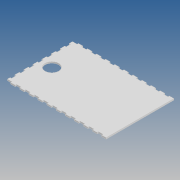
# Autodesk Inventor part: 000.104 - Cap
Saved by Autodesk Inventor 2020 (Build 240168000, 168)
## iProperties
Created: 2021-06-28
Part Number: 000.104 - Cap
Material: Типовые
Document SubType Name: Modeling
Designer: Петров Иван
Mass: 93.6094 g
Surface Area: 653.89 cm^2
Volume: 93.6094 cm^3
Density: 1 g/cm^3
Appearance: По умолчанию
Author: Петров Иван
Autodesk Inventor part; units mm, degrees
ref_plane "YZ Plane" through (0, 0, 0) normal (1, 0, 0) x (0, 1, 0)
ref_plane "XZ Plane" through (0, 0, 0) normal (0, 1, 0) x (-1, 0, 0)
ref_plane "XY Plane" through (0, 0, 0) normal (0, 0, 1) x (1, 0, 0)
sketch "Эскиз5" plane through (0, 0, 0) normal (0, 1, 0) x (-1, 0, 0)
  line L0 (-110, 74.5) -> (110, 74.5)
  line L1 (110, 74.5) -> (110, -74.5)
  line L2 (110, -74.5) -> (-110, -74.5)
  line L3 (-110, -74.5) -> (-110, 74.5)
  line L4 (-110, 74.5) -> (110, -74.5) construction
  line L5 (110, 74.5) -> (-110, -74.5) construction
  point P0 (0, 0)
  dimension "d25" = 220
  dimension "d26" = 149
  constraints: 12 end point, 2 midpoint, 2 parallel, 1 horizontal, 1 perpendicular
  measures "d25" distance of L1.end L2.end
  measures "d26" distance of L0.end L1.end
extrude "Выдавливание5" add sketch "Эскиз5" along normal blind 3
sketch "Эскиз6" plane through (0, 3, 0) normal (0, 1, 0) x (1, 0, 0)
  line L0 (-110, 74.5) -> (-110, -74.5) projected
  line L1 (-110, -65.5) -> (-107, -65.5)
  line L2 (-107, -65.5) -> (-107, -55.5)
  line L3 (-107, -55.5) -> (-110, -55.5)
  line L4 (-110, -55.5) -> (-110, -65.5)
  line L5 (-110, -74.5) -> (110, -74.5) projected
  point P0 (0, 0)
  point P1 (-107, -74.5)
  point P2 (-110, -65.5)
  dimension "d29" = 3
  dimension "d30" = 10
  dimension "d46" = 9
  constraints: 9 end point, 2 parallel, 1 perpendicular
  measures "d29" distance of L3.end L2.end
  measures "d30" distance of L2.end L1.end
  measures "d46" distance between parallel lines of L5 L1
extrude "Выдавливание6" cut sketch "Эскиз6" against normal blind 3
pattern_linear "Прямоуг.массив6" count 7 spacing 20 along (0, 0, -1) of "Выдавливание6"
sketch "Эскиз8" plane through (0, 3, 0) normal (0, 1, 0) x (1, 0, 0)
  line L0 (-110, -74.5) -> (110, -74.5) projected
  line L1 (-110, -74.5) -> (-100, -74.5)
  line L2 (-100, -74.5) -> (-100, -71.5)
  line L3 (-100, -71.5) -> (-110, -71.5)
  line L4 (-110, -71.5) -> (-110, -74.5)
  line L5 (-107, -55.5) -> (-107, -65.5) projected
  point P0 (0, 0)
  dimension "d50" = 3
  dimension "d51" = 10
  dimension "d52" = 3
  constraints: 8 end point, 2 parallel, 1 horizontal, 1 perpendicular, 1 point on line
  measures "d50" distance of L1.end L2.end
  measures "d51" distance of L2.end L3.end
  measures "d52" distance between parallel lines of L5 L4
extrude "Выдавливание8" cut sketch "Эскиз8" against normal blind 3
pattern_linear "Прямоуг.массив7" count 11 spacing 20 along (1, 0, 0) of "Выдавливание8"
mirror "Зеркальное отражение2" about plane through (0, 0, 0) normal (0, 0, 1) of "Выдавливание8", "Прямоуг.массив7"
sketch "Эскиз9" plane through (0, 3, 0) normal (0, 1, 0) x (1, 0, 0)
  circle A0 centre (-83.8133, 0) radius 15
  point P0 (0, 0)
  dimension "d58" = 30
  constraints: 1 centre point
  measures "d58" diameter of A0
extrude "Выдавливание9" cut sketch "Эскиз9" against normal blind 3
